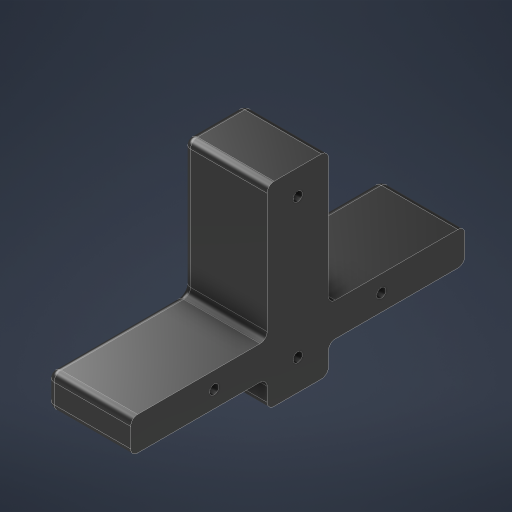
# Autodesk Inventor part: brain mount
Saved by Autodesk Inventor 2024 (Build 280153000, 153)
## iProperties
Created: 2023-12-20
Part Number: brain mount
Material: Generic
Document SubType Name: Modeling
Designer: elite
Density: 1 g/cm^3
Appearance: Glossy - Black
Author: elite
Autodesk Inventor part; units mm, degrees
ref_plane "YZ Plane" through (0, 0, 0) normal (1, 0, 0) x (0, 1, 0)
ref_plane "XZ Plane" through (0, 0, 0) normal (0, 1, 0) x (-1, 0, 0)
ref_plane "XY Plane" through (0, 0, 0) normal (0, 0, 1) x (1, 0, 0)
sketch "Sketch1" plane through (0, 0, 0) normal (1, 0, 0) x (0, 1, 0)
  line L0 (0, 0) -> (15.24, 0)
  line L1 (15.24, 0) -> (15.24, -152.4)
  line L2 (15.24, -152.4) -> (0, -152.4)
  line L3 (0, -152.4) -> (0, 0)
  line L4 (15.24, -76.2) -> (0, -76.2)
  line L5 (7.62, -76.2) -> (7.62, -114.3)
  line L6 (7.62, -76.2) -> (7.62, -38.1)
  circle A0 centre (7.62, -38.1) radius 2.1082
  circle A1 centre (7.62, -114.3) radius 2.1082
  line L7 (0, -76.2) -> (76.2, -76.2)
  line L8 (76.2, -76.2) -> (76.2, -90.17)
  line L9 (76.2, -90.17) -> (76.2, -62.23)
  line L10 (76.2, -62.23) -> (0, -62.23)
  line L11 (0, -62.23) -> (0, -90.17)
  line L12 (0, -90.17) -> (76.2, -90.17)
  line L13 (76.2, -90.17) -> (76.2, -62.23)
  line L14 (76.2, -76.2) -> (64.77, -76.2)
  circle A2 centre (64.77, -76.2) radius 2.1082
  line L15 (0, -62.23) -> (-12.7, -62.23)
  line L16 (-12.7, -62.23) -> (-12.7, -90.17)
  line L17 (-12.7, -90.17) -> (0, -90.17)
  line L18 (0, -90.17) -> (0, -62.23)
  line L19 (-12.7, -76.2) -> (1.27, -76.2)
  circle A3 centre (1.27, -76.2) radius 2.1082
  point P0 (15.24, -62.23)
  point P1 (15.24, -90.17)
  point P2 (0, -62.23)
  dimension "d0" = 152.4
  dimension "d1" = 15.24
  dimension "d2" = 38.1
  dimension "d3" = 38.1
  dimension "d4" = 4.2164
  dimension "d5" = 4.2164
  dimension "d6" = 76.2
  dimension "d7" = 13.97
  dimension "d8" = 27.94
  dimension "d12" = 11.43
  dimension "d13" = 4.2164
  dimension "d14" = 12.7
  dimension "d15" = 13.97
  dimension "d16" = 4.2164
  constraints: 40 end point, 6 parallel, 5 point on line, 4 centre point, 4 coincident, 4 midpoint, 4 perpendicular, 3 horizontal, 2 vertical
  measures "d0" distance of L2.end L0.start
  measures "d1" distance of L0.start L0.end
  measures "d2" distance of L5.start L5.end
  measures "d3" distance of L5.start L6.end
  measures "d4" diameter of A0
  measures "d5" diameter of A1
  measures "d6" distance of L4.end L7.end
  measures "d7" distance of L7.end L8.end
  measures "d8" distance of L8.end L9.end
  measures "d12" distance of L7.end L14.end
  measures "d13" diameter of A2
  measures "d14" distance of L17.end L16.end
  measures "d15" distance of L19.start L19.end
  measures "d16" diameter of A3
extrude "Extrusion1" add sketch "Sketch1" along normal blind 38.1 contours L0 L1 L10 L3 | L10 L6 L4 A3 L3 | L3 A3 L19 L16 L15 | L10 L9 L7 A2 L1 | L1 L4 L6 L10 | L7 A2 L8 L12 L1 | L1 L12 L5 L4 | L4 L5 L12 L3 A3 | A3 L3 L17 L16 L19 | L1 L2 L3 L12
fillet "Fillet1" radius 3.175 25 edges at (0, 15.24, -31.115) (0, 7.62, 0) (0, 0, -121.285) (0, 0, -31.115) (0, 7.62, -152.4) (0, 15.24, -121.285) (0, 45.72, -90.17) (0, 76.2, -69.215) (0, 76.2, -83.185) (0, 45.72, -62.23) (19.05, 15.24, 0) (19.05, 76.2, -62.23) (19.05, 15.24, -62.23) (19.05, 76.2, -90.17) (19.05, 15.24, -90.17) (19.05, 15.24, -152.4) (19.05, 0, -152.4) (19.05, 0, 0) (19.05, 0, -62.23) (19.05, -12.7, -62.23) (19.05, -12.7, -90.17) (19.05, 0, -90.17) (0, -12.7, -76.2) (0, -6.35, -62.23) (0, -6.35, -90.17)
sketch "Sketch2" plane through (0, 0, 0) normal (-1, 0, 0) x (0, 0, 1)
  circle A0 centre (-76.2, 1.27) radius 2.1082 projected
  circle A1 centre (-76.2, 1.27) radius 5.08
  circle A2 centre (-76.2, 64.77) radius 2.1082 projected
  circle A3 centre (-76.2, 64.77) radius 5.08
  point P0 (0, 0)
  dimension "d17" = 10.16
  dimension "d18" = 10.16
  constraints: 2 centre point, 2 coincident
  measures "d17" diameter of A1
  measures "d18" diameter of A3
extrude "Extrusion2" cut sketch "Sketch2" against normal blind 10.16
body "Solid1"
